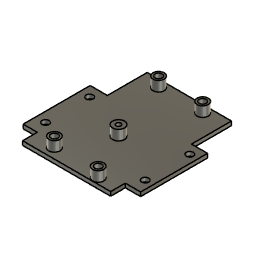
Root_Havok A1M1900X MOD 5 Universal Mount Board (Autodesk Fusion 360 design; units mm, degrees)
part number: 2025-05-15-08-56-25-947
Autodesk Fusion 360 part; units mm, degrees
sketch "Main Body" plane through (0, 0, 31) normal (0, 0, 1) x (-1, 0, 0)
  line L0 (-25.9527, 7.7965) -> (-25.9527, 47.7035)
  arc A0 (-25.9527, 47.7035) -> (-19.4062, 54.25) centre (-23.7027, 52) ccw
  line L1 (-19.4062, 54.25) -> (30.1916, 54.25)
  arc A1 (30.1916, 54.25) -> (36.7381, 47.7035) centre (34.4881, 52) ccw
  line L2 (36.7381, 47.7035) -> (36.7381, 7.7965)
  arc A2 (36.7381, 7.7965) -> (36.7381, -0.7965) centre (34.4881, 3.5) ccw
  line L3 (36.7381, -0.7965) -> (36.7381, -40.7035)
  arc A3 (36.7381, -40.7035) -> (30.4931, -42.25) centre (34.4881, -45) ccw
  line L4 (30.4931, -42.25) -> (8.822, -42.25)
  line L5 (8.822, -42.25) -> (8.822, -47.25)
  line L6 (8.822, -47.25) -> (-0.027, -47.25)
  line L7 (-0.027, -47.25) -> (-25.068, -38.1358)
  line L8 (-25.068, -38.1358) -> (-25.9527, -36.8723)
  line L9 (-25.9527, -36.8723) -> (-25.9527, -0.7965)
  arc A4 (-25.9527, -0.7965) -> (-25.9527, 7.7965) centre (-23.7027, 3.5) ccw
  circle A5 centre (34.4881, 52) radius 2.1
  circle A6 centre (34.4881, -45) radius 2.1
  circle A7 centre (-23.7027, 52) radius 2.1
  circle A8 centre (34.4881, 3.5) radius 2.1
  circle A9 centre (-23.7027, 3.5) radius 2.1
  line L10 (26.9185, -45) -> (26.9185, -50)
  line L11 (26.9185, -50) -> (37.4881, -50)
  line L12 (37.4881, -50) -> (39.4881, -48)
  line L13 (39.4881, -48) -> (39.4881, 55)
  line L14 (39.4881, 55) -> (37.4881, 57)
  line L15 (37.4881, 57) -> (-26.7027, 57)
  line L16 (-26.7027, 57) -> (-28.7027, 55)
  line L17 (-28.7027, 55) -> (-28.7027, -37.7394)
  line L18 (-28.7027, -37.7394) -> (-26.8233, -40.4234)
  line L19 (-26.8233, -40.4234) -> (-0.5119, -50)
  line L20 (-0.5119, -50) -> (11.5758, -50)
  line L21 (11.5758, -50) -> (11.5758, -45)
  line L22 (11.5758, -45) -> (26.9185, -45)
  line L23 (-24, 45) -> (-24, 11.5926)
  line L24 (-24, 11.5926) -> (-16, 11.5926)
  line L25 (-16, 11.5926) -> (-16, -8.3159)
  line L26 (-16, -8.3159) -> (26, -8.3159)
  line L27 (26, -8.3159) -> (26, 11.5926)
  line L28 (26, 11.5926) -> (34.5888, 11.5926)
  line L29 (34.5888, 11.5926) -> (34.5888, 45)
  line L30 (34.5888, 45) -> (27.5619, 45)
  line L31 (27.5619, 45) -> (27.5619, 52.3007)
  line L32 (27.5619, 52.3007) -> (-16.3603, 52.3007)
  line L33 (-16.3603, 52.3007) -> (-16.3603, 45)
  line L34 (-16.3603, 45) -> (-24, 45)
  constraint parallel L0 L23
  constraint perpendicular L23 L24
  constraint perpendicular L24 L25
  constraint perpendicular L23 L26
  constraint perpendicular L26 L27
  constraint perpendicular L23 L28
  constraint perpendicular L28 L29
  constraint perpendicular L29 L30
  constraint perpendicular L30 L31
  constraint perpendicular L29 L32
  constraint perpendicular L32 L33
  constraint perpendicular L23 L34
extrude "Extrude2" add sketch "Main Body" along normal blind 2 contours L23 L24 L25 L26 L27 L28 L29 L30 L31 L32 L33 L34
sketch "Mount Holes" plane through (0, 0, 33) normal (0, 0, 1) x (-1, 0, 0)
  line L0 (-16.3603, 45) -> (-24, 45)
  line L1 (-24, 45) -> (-24, 11.5926)
  line L2 (-24, 11.5926) -> (-16, 11.5926)
  line L3 (-16, 11.5926) -> (-16, -8.3159)
  line L4 (-16, -8.3159) -> (26, -8.3159)
  line L5 (26, -8.3159) -> (26, 11.5926)
  line L6 (26, 11.5926) -> (34.5888, 11.5926)
  line L7 (34.5888, 11.5926) -> (34.5888, 45)
  line L8 (34.5888, 45) -> (27.5619, 45)
  line L9 (27.5619, 45) -> (27.5619, 52.3007)
  line L10 (27.5619, 52.3007) -> (-16.3603, 52.3007)
  line L11 (-16.3603, 52.3007) -> (-16.3603, 45)
  circle A0 centre (-20, 16.4433) radius 1.75
  circle A1 centre (-19.9996, 38.7256) radius 1.75
  circle A2 centre (29.748, 38.6721) radius 1.75
  circle A3 centre (29.7537, 16.66) radius 1.75
  dimension "d373" = 3.5
  dimension "d374" = 3.5
  dimension "d375" = 3.5
  dimension "d376" = 3.5
  measures "d373" diameter of A0
  measures "d374" diameter of A1
  measures "d375" diameter of A2
  measures "d376" diameter of A3
extrude "Extrude3" cut sketch "Mount Holes" against normal blind 2.1 contours A0 | A1 | A2 | A3
sketch "Mount Studs" plane through (0, 0, 33) normal (0, 0, 1) x (-1, 0, 0)
  circle A0 centre (-5.3137, -4.6628) radius 2.8
  circle A1 centre (16.6535, -4.6101) radius 2.8
  circle A2 centre (16.6535, 47.3514) radius 2.8
  circle A3 centre (-7.2721, 49.4282) radius 2.8
  dimension "d379" = 5.6
  dimension "d380" = 5.6
  dimension "d381" = 5.6
  dimension "d382" = 5.6
  measures "d379" diameter of A0
  measures "d380" diameter of A1
  measures "d381" diameter of A2
  measures "d382" diameter of A3
extrude "Extrude4" add sketch "Mount Studs" along normal blind 5
sketch "Stud Heat Inserts" plane through (0, 0, 38) normal (0, 0, 1) x (-1, 0, 0)
  circle A0 centre (16.6535, 47.3514) radius 2.8
  circle A1 centre (16.6535, 47.3514) radius 1.75
  circle A2 centre (-7.2856, 49.4187) radius 1.75
  circle A3 centre (-5.3149, -4.6303) radius 1.75
  circle A4 centre (16.6535, -4.6303) radius 1.75
  dimension "d388" = 3.5
  dimension "d389" = 3.5
  dimension "d390" = 3.5
  dimension "d391" = 3.5
  constraint concentric A0 A1
  measures "d388" diameter of A1
  measures "d389" diameter of A2
  measures "d390" diameter of A3
  measures "d391" diameter of A4
extrude "Extrude5" cut sketch "Stud Heat Inserts" against normal blind 4.5 contours A1 | A2 | A3 | A4
sketch "Sketch9" plane through (0, 0, 33) normal (0, 0, 1) x (-1, 0, 0)
  circle A0 centre (5.658, 26.3539) radius 3
  circle A1 centre (5.658, 26.3539) radius 1.15
  dimension "d425" = 6
  dimension "d426" = 2.3
  constraint concentric A0 A1
  measures "d425" diameter of A0
  measures "d426" diameter of A1
extrude "Extrude6" add sketch "Sketch9" along normal blind 5 contours A0 | A1
extrude "Extrude7" cut sketch "Sketch9" against normal blind 3 contours A1
sketch "Sketch10" plane through (0, 0, 38) normal (0, 0, 1) x (-1, 0, 0)
  circle A0 centre (5.658, 26.3539) radius 3
  circle A1 centre (5.658, 26.3539) radius 1.2
  dimension "d431" = 2.4
  constraint concentric A0 A1
  measures "d431" diameter of A1
extrude "Extrude8" cut sketch "Sketch10" against normal blind 3 contours A1
